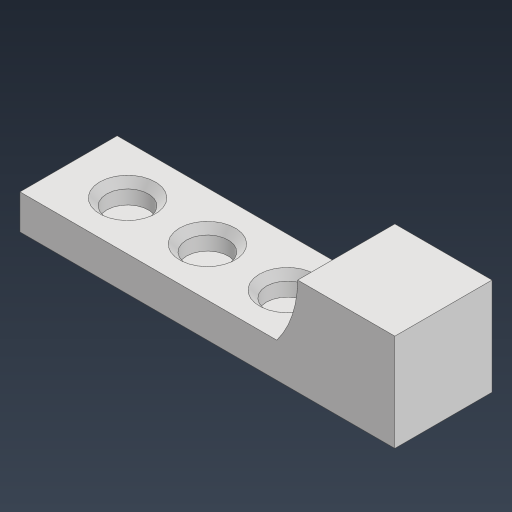
# Autodesk Inventor part: glue_test_flex
Saved by Autodesk Inventor 2023 (Build 270158000, 158)
## iProperties
Created: 2025-12-21
Part Number: glue_test_flex
Material: Generic
Document SubType Name: Modeling
Designer: szymo
Density: 1 g/cm^3
Appearance: Default
Author: szymo
Autodesk Inventor part; units mm, degrees
ref_plane "YZ Plane" through (0, 0, 0) normal (1, 0, 0) x (0, 1, 0)
ref_plane "XZ Plane" through (0, 0, 0) normal (0, 1, 0) x (-1, 0, 0)
ref_plane "XY Plane" through (0, 0, 0) normal (0, 0, 1) x (1, 0, 0)
sketch "Sketch1" plane through (0, 0, 0) normal (0, 1, 0) x (-1, 0, 0)
  line L0 (-13.5, -3.5) -> (13.5, -3.5)
  line L1 (13.5, -3.5) -> (13.5, 3.5)
  line L2 (13.5, 3.5) -> (-13.5, 3.5)
  line L3 (-13.5, 3.5) -> (-13.5, -3.5)
  line L4 (-13.5, -3.5) -> (13.5, 3.5) construction
  line L5 (13.5, -3.5) -> (-13.5, 3.5) construction
  line L6 (-6.5, 3.5) -> (-6.5, -3.5)
  line L7 (-6.5, 0) -> (13.5, 0) construction
  circle A0 centre (9.25, 0) radius 1.5
  circle A1 centre (3.5, 0) radius 1.5
  circle A2 centre (-2.25, 0) radius 1.5
  point P0 (0, 0)
  dimension "d0" = 27
  dimension "d1" = 7
  dimension "d2" = 7
  dimension "d3" = 3
  dimension "d6" = 3
  dimension "d11" = 3
  dimension "d19" = 5.75
  dimension "d20" = 5.75
  dimension "d21" = 4.25
  dimension "d22" = 4.25
  constraints: 16 end point, 5 midpoint, 4 point on line, 3 centre point, 2 parallel, 2 perpendicular, 1 horizontal
  measures "d0" distance of L2.end L1.end
  measures "d1" distance of L1.end L0.end
  measures "d2" distance between parallel lines of L3 L6
  measures "d3" diameter of A0
  measures "d6" diameter of A1
  measures "d11" diameter of A2
  measures "d19" distance of A2.centre A1.centre
  measures "d20" distance of A0.centre A1.centre
  measures "d21" distance from line of L6 A2.centre
  measures "d22" distance from line of L1 A0.centre
extrude "Extrusion1" add sketch "Sketch1" along normal blind 7 contours L3 L2 L6 L0
extrude "Extrusion2" add sketch "Sketch1" along normal blind 2.5 contours L6 L2 L1 L0
extrude "Extrusion3" add sketch "Sketch1" along normal blind 1 contours A0 | A1 | A2
chamfer "Chamfer1" distance 0.5 angle 45 3 edges at (3.75, 2.5, 0) (-2, 2.5, 0) (-7.75, 2.5, 0)
sketch "Sketch2" plane through (13.5, 7, -3.5) normal (0, 0, -1) x (-1, 0, 0)
  line L0 (0, -7) -> (27, -7) projected
  line L1 (27, -7) -> (27, -4.5) projected
  line L2 (7, -4.5) -> (27, -4.5) projected
  line L3 (7, -4.5) -> (7, 0) projected
  line L4 (0, 0) -> (7, 0) projected
  line L5 (0, -7) -> (0, 0) projected
  arc A0 (7, 0) -> (8.5, -4.5) centre (14.5, 0) ccw
  point P0 (13.5, -7)
  dimension "d32" = 1.5
  constraints: 2 point on circle, 1 centre point, 1 point on line, 1 tangent
  measures "d32" distance of L2.start A0.end
extrude "Extrusion4" add sketch "Sketch2" against normal up to surface (7 mm away) contours A0 L2 L3
equation "\"d20\" = d19"
equation "\"d21\" = d19 - 0.5 * d11"
equation "\"d22\" = d19 - 0.5 * d3"
body "Solid1"
